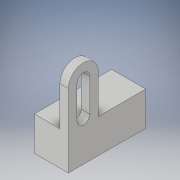
# Autodesk Inventor part: 17 slot tegen pin
Saved by Autodesk Inventor 2019 (Build 230136000, 136)
## iProperties
Created: 2021-01-19
Part Number: 17 slot tegen pin
Material: Generic
Document SubType Name: Modeling
Designer: Stefan
Density: 1 g/cm^3
Appearance: Default
Author: Stefan
Autodesk Inventor part; units mm, degrees
ref_plane "YZ Plane" through (0, 0, 0) normal (1, 0, 0) x (0, 1, 0)
ref_plane "XZ Plane" through (0, 0, 0) normal (0, 1, 0) x (-1, 0, 0)
ref_plane "XY Plane" through (0, 0, 0) normal (0, 0, 1) x (1, 0, 0)
sketch "Sketch1" plane through (0, 0, 0) normal (0, 0, 1) x (1, 0, 0)
  line L0 (-6, -6) -> (6, -6)
  line L1 (6, -6) -> (6, 6)
  line L2 (6, 6) -> (-6, 6)
  line L3 (-6, 6) -> (-6, -6)
  line L4 (-6, -6) -> (6, 6) construction
  line L5 (6, -6) -> (-6, 6) construction
  point P0 (0, 0)
  dimension "d0" = 12
  dimension "d1" = 12
  constraints: 12 end point, 2 midpoint, 2 parallel, 1 horizontal, 1 perpendicular
  measures "d0" distance of L2.end L1.end
  measures "d1" distance of L1.end L0.end
extrude "Extrusion1" add sketch "Sketch1" along normal blind 27.2
sketch "Sketch2" plane through (6, -6, 0) normal (1, 0, 0) x (0, 0, -1)
  arc A0 (-24.2, 14.25) -> (-19.7, 14.25) centre (-21.95, 14.25) ccw
  line L0 (-27.2, 0) -> (-27.2, 12) projected
  line L1 (0, 12) -> (-27.2, 12) projected
  line L2 (-21.95, 14.25) -> (-21.95, 25.75) construction
  arc A1 (-19.7, 25.75) -> (-24.2, 25.75) centre (-21.95, 25.75) ccw
  line L3 (-24.2, 25.75) -> (-24.2, 14.25)
  line L4 (-19.7, 25.75) -> (-19.7, 14.25)
  arc A2 (-16.7, 25.75) -> (-27.2, 25.75) centre (-21.95, 25.75) ccw
  line L5 (-16.7, 25.75) -> (-16.7, 12)
  line L6 (-27.2, 25.75) -> (-27.2, 12)
  line L7 (-27.2, 12) -> (-27.2, 12)
  point P0 (0, 6)
  dimension "d4" = 4.5
  dimension "d5" = 5.25
  dimension "d6" = 2.25
  dimension "d7" = 11.5
  dimension "d8" = 4.5
  dimension "d9" = 10.5
  dimension "d10" = 13.75
  constraints: 12 end point, 6 point on circle, 5 tangent, 3 centre point, 2 coincident, 2 perpendicular, 2 vertical, 1 point on line
  measures "d4" diameter of A0
  measures "d5" distance from line of L0 L2.start
  measures "d6" distance from line of L1 L2.start
  measures "d7" distance of L2.start L2.end
  measures "d8" diameter of A1
  measures "d9" diameter of A2
  measures "d10" distance of L5.start L5.end
extrude "Extrusion2" add sketch "Sketch2" against normal blind 3
body "Solid1"
